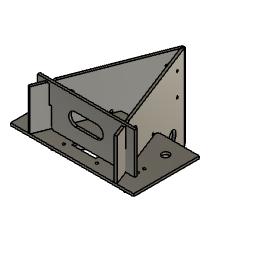
2425-SACBOT-LINEv6 (Autodesk Fusion 360 design; units mm, degrees)
Autodesk Fusion 360 part; units mm, degrees
sketch "Plate Alpha" plane through (0, 0, 0) normal (0, 0, 1) x (1, 0, 0)
  line L0 (-51.3733, 27.0083) -> (98.6267, 27.0083)
  line L1 (98.6267, 27.0083) -> (98.6267, -52.9917)
  line L2 (98.6267, -52.9917) -> (-51.3733, -52.9917)
  line L3 (-51.3733, -52.9917) -> (-51.3733, 27.0083)
  circle A0 centre (-31.3733, -27.9917) radius 1.5
  circle A1 centre (-31.3733, -19.9917) radius 1.5
  line L4 (23.6267, 82.9359) -> (-12.5865, -10.2768)
  line L5 (22.2285, 83.4791) -> (-13.9847, -9.7336)
  line L6 (25.0248, 82.3927) -> (-11.1883, -10.82)
  line L7 (23.6267, 27.0083) -> (23.6267, -52.9917) construction
  line L8 (-13.9847, -9.7336) -> (-11.1883, -10.82)
  circle A2 centre (3.4767, -42.9917) radius 1.5
  circle A3 centre (3.4767, -17.4917) radius 1.5
  line L9 (98.6267, -52.9917) -> (98.6267, 27.0083)
  circle A4 centre (78.6267, -27.9917) radius 1.5
  circle A5 centre (43.7767, -42.9917) radius 1.5
  circle A6 centre (78.6267, -19.9917) radius 1.5
  line L10 (23.6267, 82.9359) -> (59.8398, -10.2768)
  circle A7 centre (43.7767, -17.4917) radius 1.5
  line L11 (22.2285, 82.3927) -> (58.4416, -10.82)
  line L12 (61.238, -9.7336) -> (58.4416, -10.82)
  line L13 (25.0248, 83.4791) -> (61.238, -9.7336)
  line L14 (23.6267, 27.0083) -> (23.6267, 163.1815)
  line L15 (-31.3733, -27.9917) -> (-31.3733, -19.9917) construction
  line L16 (3.4767, -42.9917) -> (3.4767, -17.4917) construction
  line L17 (-12.5865, -10.2768) -> (-29.1813, -52.9917) construction
  line L18 (-51.3733, -32.8941) -> (98.6267, -32.8941) construction
  arc A8 (5.5609, 27.0083) -> (2.7645, 25.0947) centre (5.5609, 24.0083) ccw
  arc A9 (-1.298, 22.9219) -> (-4.0944, 27.0083) centre (-4.0944, 24.0083) ccw
  arc A10 (51.3477, 27.0083) -> (48.5513, 22.9219) centre (51.3477, 24.0083) ccw
  arc A11 (44.4888, 25.0947) -> (41.6924, 27.0083) centre (41.6924, 24.0083) ccw
  line L19 (3.4766, -15.9917) -> (-5.5103, -15.9917)
  line L20 (-5.5103, -15.9917) -> (43.7767, -15.9917)
  line L21 (1.9767, -17.4917) -> (1.9767, -42.9917)
  line L22 (3.4767, -44.4917) -> (43.7767, -44.4917)
  line L23 (9.2267, -17.4917) -> (9.2267, -42.9917)
  line L24 (3.4767, -38.9917) -> (43.7767, -38.9917)
  line L25 (38.0267, -17.4917) -> (38.0267, -42.9917)
  line L26 (-51.3733, 7.77) -> (98.6267, 7.77) construction
  line L27 (-29.6655, 27.0083) -> (-29.6655, -14.5276) construction
  line L28 (3.4766, -8.7417) -> (-5.5103, -8.7417)
  arc A12 (-5.5103, -8.7417) -> (-5.5103, -23.2417) centre (-5.5103, -15.9917) ccw
  line L29 (-5.5103, -23.2417) -> (43.7767, -23.2417)
  circle A13 centre (-29.6655, 7.77) radius 4.5
  circle A14 centre (76.9188, 7.77) radius 4.5
  point P0 (1.8988, 27.0083)
  point P1 (45.3545, 27.0083)
  point P2 (47.2533, 0)
  point P3 (-21.3733, -32.8941)
  dimension "d1" = 1.5
  dimension "d2" = -1.5
  dimension "d3" = 75
  dimension "d4" = 3
  dimension "d5" = 3
  dimension "d6" = 8
  dimension "d7" = 20
  dimension "d9" = 40
  dimension "d10" = 80
  dimension "d11" = 25.5
  dimension "d12" = 3
  dimension "d13" = 3
  dimension "d14" = 10
  dimension "d15" = 20.15
  dimension "d16" = 60
  dimension "d35" = 25
  dimension "d38" = 45
  dimension "d62" = 3
  dimension "d63" = 3
  dimension "d76" = 7.25
  dimension "d77" = -7.25
  dimension "d78" = -5.5
  dimension "d79" = 9
  constraint horizontal L0
  constraint vertical L1
  constraint horizontal L2
  constraint vertical L3
  constraint midpoint L0 L7.start
  constraint midpoint L2 L7.end
  constraint coincident L0 P0
  constraint coincident L4 P0
  constraint perpendicular L6 L8
  constraint symmetric origin L7 P2
  constraint symmetric L0.start L7 L0.end
  constraint symmetric L2.end L7 L1.end
  constraint symmetric A0 L7 A4
  constraint symmetric A1 L7 A6
  constraint symmetric L4.start L7 L10.start
  constraint symmetric L4.end L7 L10.end
  constraint symmetric L5.start L7 L13.start
  constraint symmetric L5.end L7 L12.start
  constraint symmetric L6.start L7 L11.start
  constraint symmetric L6.end L7 L11.end
  constraint symmetric L7 P0 P1
  constraint symmetric L7 A2 A5
  constraint symmetric L7 A3 A7
  constraint perpendicular L0 L14
  constraint coincident L4.start L14
  constraint coincident A0.centre L15.start
  constraint coincident A1.centre L15.end
  constraint coincident A2.centre L16.start
  constraint coincident A3.centre L16.end
  constraint vertical L16
  constraint vertical L15
  constraint coincident L2 L17.end
  constraint parallel L6 L17
  constraint coincident L3 L18.start
  constraint coincident L1 L18.end
  constraint perpendicular L1 L18
  constraint coincident L17 P3
  constraint coincident L18 P3
  constraint tangent L6 A8
  constraint tangent L0 A8
  constraint coincident L6 A8.end
  constraint coincident L0 A8.start
  constraint tangent L0 A9
  constraint tangent L5 A9
  constraint coincident L0 A9.end
  constraint coincident L5 A9.start
  constraint symmetric L7 A8.end A11.start
  constraint symmetric L7 A8.start A11.end
  constraint symmetric L7 A8 A11
  constraint symmetric L7 A9.end A10.start
  constraint symmetric L7 A9.start A10.end
  constraint symmetric L7 A9 A10
  constraint horizontal L19
  constraint tangent A3 L20
  constraint tangent A7 L20
  constraint coincident A3 L19.start
  constraint coincident A7 L20.end
  constraint coincident A3 L21.start
  constraint tangent A3 L21
  constraint coincident A2 L21.end
  constraint tangent A2 L21
  constraint coincident A2 L22.start
  constraint coincident A5 L22.end
  constraint tangent A2 L22
  constraint tangent A5 L22
  constraint symmetric L7 L23.start L25.start
  constraint symmetric L7 L23.end L25.end
  constraint coincident L3 L26.start
  constraint coincident L1 L26.end
  constraint perpendicular L1 L26
  constraint coincident L0 L27.start
  constraint perpendicular L0 L27
  constraint coincident L26 A13.centre
  constraint coincident L27 A13.centre
  constraint symmetric L7 A13 A14
  measures "d3" distance of L3 L7
  measures "d4" diameter of A0
  measures "d5" diameter of A1
  measures "d6" vertical distance of A0.centre A1.centre
  measures "d7" distance of L3 A0.centre
  measures "d9" distance of L4.end P0
  measures "d10" distance of L0.start L2.end
  measures "d11" distance of A2.centre A3.centre
  measures "d12" diameter of A2
  measures "d13" diameter of A3
  measures "d14" distance of L2 A2.centre
  measures "d15" distance of L7 A2.centre
  measures "d16" distance of L4.start P0
  measures "d35" distance of L2 A0.centre
  measures "d38" distance of L7 P3
  measures "d62" radius of A8
  measures "d63" radius of A9
  measures "d79" diameter of A13
sketch "Plate Beta" plane through (0, 0, 0) normal (0, 0, 1) x (1, 0, 0)
  line L0 (42.32, -117.937) -> (42.32, -67.937)
  line L1 (42.32, -67.937) -> (187.82, -67.937)
  line L2 (187.82, -67.937) -> (187.82, -169.0723)
  line L3 (184.0759, -171.9785) -> (62.82, -140.937)
  line L4 (62.82, -140.937) -> (62.82, -117.937)
  line L5 (62.82, -117.937) -> (42.32, -117.937)
  line L6 (62.82, -67.937) -> (62.82, -92.937)
  line L7 (60.62, -67.937) -> (60.62, -92.937)
  line L8 (65.02, -67.937) -> (65.02, -92.937)
  line L9 (60.62, -92.937) -> (65.02, -92.937)
  line L10 (62.82, -117.937) -> (87.82, -117.937)
  line L11 (87.82, -117.937) -> (87.82, -120.937)
  line L12 (87.82, -120.937) -> (62.82, -120.937)
  line L13 (23.6267, 82.9359) -> (59.8398, -10.2768)
  line L14 (-51.3733, 27.0083) -> (98.6267, 27.0083)
  arc A0 (60.62, -70.937) -> (57.62, -67.937) centre (57.62, -70.937) ccw
  arc A1 (68.02, -67.937) -> (65.02, -70.937) centre (68.02, -70.937) ccw
  arc A2 (65.82, -120.937) -> (62.82, -123.937) centre (65.82, -123.937) ccw
  arc A3 (184.0759, -171.9785) -> (187.82, -169.0723) centre (184.82, -169.0723) ccw
  line L15 (79.6707, -67.937) -> (79.6707, -104.5478) construction
  line L16 (79.6707, -86.2424) -> (95.5231, -86.2424) construction
  line L17 (95.5231, -86.2424) -> (145.91, -86.2424) construction
  circle A4 centre (79.6707, -86.2424) radius 4.5
  line L18 (105.02, -57.3516) -> (105.02, -183.7559) construction
  line L19 (87.82, -117.937) -> (187.82, -117.937) construction
  line L20 (119.02, -57.3516) -> (119.02, -183.7559) construction
  line L21 (171.12, -57.3516) -> (171.12, -183.7559) construction
  line L22 (87.82, -115.437) -> (187.82, -115.437) construction
  line L23 (87.82, -110.337) -> (187.82, -110.337) construction
  line L24 (87.82, -82.437) -> (187.82, -82.437) construction
  circle A5 centre (119.02, -115.437) radius 1.5
  circle A6 centre (171.12, -110.337) radius 1.5
  circle A7 centre (171.12, -82.437) radius 1.5
  circle A8 centre (159.8734, -146.2859) radius 8
  point P0 (187.82, -172.937)
  dimension "d17" = 2.2
  dimension "d18" = -2.2
  dimension "d19" = 25
  dimension "d20" = 50
  dimension "d21" = 3
  dimension "d22" = 25
  dimension "d25" = 20.5
  dimension "d26" = 20.5
  dimension "d27" = 100
  dimension "d28" = 20
  dimension "d36" = 55
  dimension "d64" = 3
  dimension "d65" = 6
  dimension "d66" = 3
  dimension "d67" = 3
  dimension "d80" = 9
  dimension "d81" = 40
  dimension "d82" = -14
  dimension "d83" = -66.1
  dimension "d84" = -2.5
  dimension "d85" = -7.6
  dimension "d86" = -35.5
  dimension "d87" = 3
  dimension "d88" = 3
  dimension "d89" = 3
  dimension "d90" = 16
  constraint vertical L0
  constraint perpendicular L0 L1
  constraint perpendicular L1 L2
  constraint parallel L2 L4
  constraint horizontal L5
  constraint coincident L1 L6.start
  constraint perpendicular L1 L6
  constraint perpendicular L8 L9
  constraint perpendicular L4 L10
  constraint perpendicular L10 L11
  constraint coincident L4 L12.end
  constraint horizontal L12
  constraint tangent L1 A0
  constraint tangent L7 A0
  constraint coincident L1 A0.end
  constraint coincident L7 A0.start
  constraint tangent L8 A1
  constraint tangent L1 A1
  constraint coincident L8 A1.end
  constraint coincident L1 A1.start
  constraint tangent L4 A2
  constraint tangent L12 A2
  constraint coincident L4 A2.end
  constraint coincident L12 A2.start
  constraint coincident P0 L3
  constraint coincident P0 L2
  constraint tangent L3 A3
  constraint tangent L2 A3
  constraint coincident L1 L15.start
  constraint perpendicular L1 L15
  constraint midpoint L15 L16.start
  constraint perpendicular L15 L16
  constraint perpendicular L15 L17
  constraint coincident L16.start A4.centre
  constraint vertical L18
  constraint coincident L2 L19.end
  constraint horizontal L19
  constraint coincident L20 A5.centre
  constraint coincident L22 A5.centre
  constraint coincident L23 A6.centre
  constraint coincident L21 A6.centre
  constraint coincident L24 A7.centre
  constraint coincident L21 A7.centre
  measures "d19" distance of L6.start L6.end
  measures "d20" distance of L0.start L0.end
  measures "d21" distance of L10.end L11.end
  measures "d22" distance of L11.end L12.end
  measures "d25" distance of L0.start L4.end
  measures "d26" distance of L0 L6
  measures "d27" distance of L2 L10.end
  measures "d28" distance of L3.end L12.end
  measures "d36" distance of P0 L10
  measures "d64" radius of A0
  measures "d65" diameter of A1
  measures "d66" radius of A2
  measures "d67" radius of A3
  measures "d80" diameter of A4
  measures "d81" distance of L8 L18
  measures "d87" diameter of A5
  measures "d88" diameter of A6
  measures "d89" diameter of A7
  measures "d90" diameter of A8
sketch "Plate Gamma" plane through (0, 0, 0) normal (0, 0, 1) x (1, 0, 0)
  line L0 (-88.0165, -70.6703) -> (30.4835, -70.6703)
  line L1 (30.4835, -70.6703) -> (30.4835, -120.6703)
  line L2 (30.4835, -120.6703) -> (-88.0165, -120.6703)
  line L3 (-88.0165, -120.6703) -> (-88.0165, -70.6703)
  line L4 (-28.7665, -70.6703) -> (-28.7665, -120.6703) construction
  circle A0 centre (-41.7665, -95.6703) radius 8
  line L5 (-41.7665, -87.6703) -> (-28.7665, -87.6703)
  line L6 (-41.7665, -103.6703) -> (-28.7665, -103.6703)
  line L7 (-73.0165, -120.6703) -> (-73.0165, -95.6703)
  line L8 (-70.8165, -120.6703) -> (-70.8165, -95.6703)
  line L9 (-75.2165, -120.6703) -> (-75.2165, -95.6703)
  line L10 (-75.2165, -95.6703) -> (-70.8165, -95.6703)
  line L11 (-88.0165, -95.6703) -> (30.4835, -95.6703) construction
  circle A1 centre (-15.7665, -95.6703) radius 8
  line L12 (-15.7665, -87.6703) -> (-28.7665, -87.6703)
  line L13 (-15.7665, -103.6703) -> (-28.7665, -103.6703)
  line L14 (13.2835, -120.6703) -> (13.2835, -95.6703)
  line L15 (17.6835, -120.6703) -> (17.6835, -95.6703)
  line L16 (17.6835, -95.6703) -> (13.2835, -95.6703)
  arc A2 (-70.8165, -117.6703) -> (-67.8165, -120.6703) centre (-67.8165, -117.6703) ccw
  arc A3 (-78.2165, -120.6703) -> (-75.2165, -117.6703) centre (-78.2165, -117.6703) ccw
  arc A4 (10.2835, -120.6703) -> (13.2835, -117.6703) centre (10.2835, -117.6703) ccw
  arc A5 (17.6835, -117.6703) -> (20.6835, -120.6703) centre (20.6835, -117.6703) ccw
  dimension "d29" = 2.2
  dimension "d30" = -2.2
  dimension "d31" = 16
  dimension "d32" = 25
  dimension "d33" = 13
  dimension "d34" = 44.25
  dimension "d39" = 15
  dimension "d68" = 3
  dimension "d69" = 6
  constraint horizontal L0
  constraint vertical L1
  constraint horizontal L2
  constraint vertical L3
  constraint midpoint L0 L4.start
  constraint midpoint L2 L4.end
  constraint coincident A0 L5.start
  constraint coincident L4 L5.end
  constraint horizontal L5
  constraint tangent A0 L5
  constraint coincident A0 L6.start
  constraint coincident L4 L6.end
  constraint horizontal L6
  constraint tangent A0 L6
  constraint coincident L2 L7.start
  constraint perpendicular L2 L7
  constraint perpendicular L8 L10
  constraint midpoint L3 L11.start
  constraint midpoint L1 L11.end
  constraint coincident A0.centre L11
  constraint coincident L7.end L11
  constraint symmetric L4 A0 A1
  constraint symmetric L4 L5.start L12.start
  constraint symmetric L4 L5.end L12.end
  constraint symmetric L4 L6.start L13.start
  constraint symmetric L4 L6.end L13.end
  constraint symmetric L4 L8.start L14.start
  constraint symmetric L4 L8.end L14.end
  constraint symmetric L4 L9.start L15.start
  constraint symmetric L4 L9.end L15.end
  constraint tangent L2 A2
  constraint tangent L8 A2
  constraint coincident L2 A2.end
  constraint coincident L8 A2.start
  constraint tangent L2 A3
  constraint tangent L9 A3
  constraint coincident L9 A3.end
  constraint coincident L2 A3.start
  constraint symmetric L4 A2.end A4.start
  constraint symmetric L4 A2.start A4.end
  constraint symmetric L4 A2 A4
  constraint symmetric L4 A3.end A5.start
  constraint symmetric L4 A3.start A5.end
  constraint symmetric L4 A3 A5
  measures "d31" diameter of A0
  measures "d32" distance of L2 A0.centre
  measures "d33" distance of L4 A0.centre
  measures "d34" distance of L4 L7.start
  measures "d39" distance of L7.end L11.start
  measures "d68" radius of A2
  measures "d69" diameter of A3
extrude "Extrude2" add sketch "Plate Alpha" along normal blind 3 contours L0 L1 L2 L3 L5 L6 L8 L9 L11 L12 L13 A8 A9 A10 A11 makes body 1
extrude "Extrude3" add sketch "Plate Beta" along normal blind 3 separate body contours L0 L1 L2 L3 L4 L5 L7 L8 L9 L10 L11 L12 A0 A1 A2 A3 makes body 2
extrude "Extrude4" add sketch "Plate Gamma" along normal blind 3 separate body contours L0 L1 L2 L3 L8 L9 L10 L14 L15 L16 A2 A3 A4 A5 makes body 3
copy_body "Body->Comp2" bodies 1 removing the originals makes body 4 in component "MainBody"
copy_body "Body->Comp3" bodies 2 removing the originals makes body 5 in component "VerticalFin/Tail"
copy_body "Body->Comp4" bodies 3 removing the originals makes body 6 in component "VerticalFront"
component "MainBody" placed x (1, 0, 0) y (0, 1, 0) z (0, 0, 1) at (0, 0, 0)
component "VerticalFin/Tail" placed x (-0.362132, 0.932127, 0) y (0, 0, 1) z (0.932127, 0.362132, 0) at (90.244, -92.6793, 120.937)
component "VerticalFront" placed x (1, -0.000544, 0) y (0, 0, 1) z (-0.000544, -1, 0) at (51.3775, -32.1197, 123.6703)
component "VerticalFin/Tail" placed x (0.362132, 0.932127, 0) y (0, 0, 1) z (0.932127, -0.362132, 0) at (-45.7871, -91.5929, 120.937)
equation "d1 = ( 3 / 2 ) * 1 mm"
equation "d2 = -1 * d1"
equation "d5 = d4"
equation "d12 = d4"
equation "d13 = d12"
equation "d20 = 2 * d19"
equation "d21 = 2 * d1"
equation "d27 = d16 + d9"
equation "d32 = d19"
equation "d33 = ( 42 mm - d31 ) / 2"
equation "d83 = -14 mm - 1.3 mm - 50.8 mm"
equation "d85 = -2.5 mm - 5.1 mm"
equation "d86 = -2.5 mm - 5.1 mm - 27.9 mm"
